Autodesk Inventor part; units mm, degrees
(part 2 of 2)
sketch "Sketch2" plane through (0, 0, 3) normal (0, 0, 1) x (1, 0, 0)
  arc A0 (-420.3678, -42.3519) -> (-416.8322, -42.3519) centre (-418.6, -40.5842) ccw projected
  line L0 (-416.8322, -42.3519) -> (-364.6059, 9.8744) projected
  arc A1 (-364.6059, 9.8744) -> (-363.8737, 11.6421) centre (-366.3737, 11.6421) ccw projected
  line L1 (-363.8737, 11.6421) -> (-363.8737, 21.1698) projected
  arc A2 (-363.8737, 21.1698) -> (-364.287, 22.5467) centre (-366.3737, 21.1698) ccw projected
  line L2 (-364.287, 22.5467) -> (-369.9099, 31.0681) projected
  arc A3 (-369.9099, 31.0681) -> (-369.9649, 31.1498) centre (-374.15, 28.2703) ccw projected
  arc A4 (-369.9649, 31.1498) -> (-372.0245, 32.2327) centre (-372.0245, 29.7327) ccw projected
  line L3 (-372.0245, 32.2327) -> (-376.3363, 32.2327) projected
  arc A5 (-376.3363, 32.2327) -> (-378.104, 31.5005) centre (-376.3363, 29.7327) ccw projected
  line L4 (-378.104, 31.5005) -> (-390.4421, 19.1624) projected
  arc A6 (-390.4421, 19.1624) -> (-391.93, 15.5703) centre (-386.85, 15.5703) ccw projected
  line L5 (-391.93, 15.5703) -> (-391.93, 4.385) projected
  arc A7 (-399.3695, -13.5755) -> (-391.93, 4.385) centre (-417.33, 4.385) ccw projected
  line L6 (-399.3695, -13.5755) -> (-422.4891, -36.6951) projected
  arc A8 (-422.4891, -36.6951) -> (-422.4891, -40.2306) centre (-420.7213, -38.4628) ccw projected
  line L7 (-422.4891, -40.2306) -> (-420.3678, -42.3519) projected
  arc A9 (-368.1126, 9.8325) -> (-370.3046, 12.0246) centre (-369.2086, 10.9286) ccw projected
  line L8 (-368.1126, 9.8325) -> (-381.583, -3.6378) projected
  arc A10 (-383.775, -1.4458) -> (-381.583, -3.6378) centre (-382.679, -2.5418) ccw projected
  line L9 (-383.775, -1.4458) -> (-370.3046, 12.0246) projected
  circle A11 centre (-391.6592, -11.5221) radius 2.159 projected
  arc A12 (-419.696, -37.3668) -> (-417.504, -39.5589) centre (-418.6, -38.4628) ccw projected
  line L10 (-419.696, -37.3668) -> (-401.7355, -19.4063) projected
  arc A13 (-399.5435, -21.5984) -> (-401.7355, -19.4063) centre (-400.6395, -20.5023) ccw projected
  line L11 (-399.5435, -21.5984) -> (-417.504, -39.5589) projected
  circle A14 centre (-380.5, 21.9203) radius 2.159 projected
  circle A15 centre (-386.85, 15.5703) radius 2.159 projected
  circle A16 centre (-374.15, 28.2703) radius 2.159 projected
  line L12 (-372.293, 29.2327) -> (-366.8737, 21.0197)
  line L13 (-366.8737, 21.0197) -> (-366.8737, 11.8492)
  line L14 (-366.8737, 11.8492) -> (-418.6, -39.8771)
  line L15 (-418.6, -39.8771) -> (-420.0142, -38.4628)
  line L16 (-420.0142, -38.4628) -> (-397.2482, -15.6968)
  arc A17 (-397.2482, -15.6968) -> (-388.93, 4.385) centre (-417.33, 4.385) ccw
  line L17 (-388.93, 4.385) -> (-388.93, 15.5703)
  arc A18 (-388.3208, 17.0411) -> (-388.93, 15.5703) centre (-386.85, 15.5703) ccw
  line L18 (-388.3208, 17.0411) -> (-376.1292, 29.2327)
  line L19 (-376.1292, 29.2327) -> (-372.293, 29.2327)
  arc A19 (-365.9913, 7.7112) -> (-372.4259, 14.1459) centre (-369.2086, 10.9286) ccw
  line L20 (-365.9913, 7.7112) -> (-379.4616, -5.7592)
  arc A20 (-385.8963, 0.6755) -> (-379.4616, -5.7592) centre (-382.679, -2.5418) ccw
  line L21 (-385.8963, 0.6755) -> (-372.4259, 14.1459)
  circle A21 centre (-391.6592, -11.5221) radius 5.159
  circle A22 centre (-386.85, 15.5703) radius 5.159
  circle A23 centre (-380.5, 21.9203) radius 5.159
  circle A24 centre (-374.15, 28.2703) radius 5.159
  circle A25 centre (-387.2958, 1.7447) radius 1.75
  point P0 (0, 0)
  point P1 (-366.8737, 14.8338)
  point P2 (-369.8137, 25.4753)
  point P3 (-375.5286, 23.2989)
  point P4 (-381.8786, 16.9489)
  point P5 (-388.93, 10.8492)
  point P6 (-389.0391, 1.898)
  point P7 (-386.0134, 0.554)
  dimension "d15" = 3
  dimension "d16" = 3
  dimension "d17" = 3
  dimension "d18" = 3
  dimension "d19" = 3.5
  constraints: 20 end point, 9 centre point, 8 point on circle, 2 coincident, 2 equal radius, 2 tangent, 12 other
  measures "d15" distance between parallel lines of L2 L12
  measures "d16" distance between parallel lines of L9 L21
  measures "d17" radial gap between concentric circles of A11 A21
  measures "d18" radial gap between concentric circles of A15 A22
  measures "d19" diameter of A25
extrude "Extrusion2" cut sketch "Sketch2" against normal blind 2 contours A19 L21 A20 A25 A17 L17 A22 A23 A24 L12 L13 | A25
fillet "Fillet3" radius 1.75 6 edges at (-366.8737, 21.0197, 2) (-366.8737, 14.8338, 2) (-369.8137, 25.4753, 2) (-375.5286, 23.2989, 2) (-381.8786, 16.9489, 2) (-388.93, 10.8492, 2)
body "Solid1"
